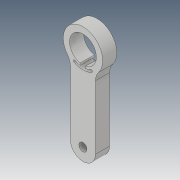
# Autodesk Inventor part: gripperPart4
Saved by Autodesk Inventor 2018 (Build 220112000, 112)
## iProperties
Created: 2020-01-19
Part Number: gripperPart4
Material: Generic
Document SubType Name: Modeling
Designer: anirudh
Density: 1 g/cm^3
Appearance: Default
Author: anirudh
Autodesk Inventor part; units mm, degrees
ref_plane "YZ Plane" through (0, 0, 0) normal (1, 0, 0) x (0, 1, 0)
ref_plane "XZ Plane" through (0, 0, 0) normal (0, 1, 0) x (-1, 0, 0)
ref_plane "XY Plane" through (0, 0, 0) normal (0, 0, 1) x (1, 0, 0)
sketch "Sketch1" plane through (0, 0, 0) normal (0, 0, 1) x (1, 0, 0)
  arc A0 (9.753, 1.6889) -> (9.316, 0.7861) centre (9.5674, 1.2216) ccw
  arc A1 (9.8188, 1.6571) -> (9.316, 0.7861) centre (9.5674, 1.2216) ccw
  arc A2 (17.316, 0.7861) -> (16.816, 1.6522) centre (17.066, 1.2191) ccw
  arc A3 (17.316, 0.7861) -> (16.816, 1.6522) centre (17.066, 1.2191) ccw
  arc A4 (14.5598, 0.8257) -> (16.816, 1.6522) centre (13.316, 7.7143) ccw
  arc A5 (9.316, 0.7861) -> (17.316, 0.7861) centre (13.316, 7.7143) ccw
  arc A6 (9.316, 0.7861) -> (17.316, 0.7861) centre (13.316, 7.7143) ccw
  arc A7 (9.8188, 1.6571) -> (12.0792, 0.8302) centre (13.316, 7.7143) ccw
  arc A8 (14.5598, 0.8257) -> (16.816, 1.6522) centre (13.316, 7.7143) ccw
  line L0 (7.6645, -17.6857) -> (7.6645, 0.8519)
  line L1 (18.9675, -17.6857) -> (18.9675, 0.8519)
  arc A9 (9.316, 0.7861) -> (17.316, 0.7861) centre (13.316, 7.7143) ccw
  line L2 (7.6645, -17.6857) -> (7.6645, -30.3857)
  line L3 (18.9675, -17.6857) -> (18.9675, -30.3857)
  arc A10 (7.6645, -30.3857) -> (18.9675, -30.3857) centre (13.316, -30.3857) ccw
  circle A11 centre (13.316, -30.3857) radius 1.8
  arc A12 (14.5512, 1.7918) -> (12.0808, 1.7918) centre (13.316, 7.7143) ccw
  arc A13 (18.9675, 0.8519) -> (7.6645, 0.8519) centre (13.316, 7.7143) ccw
  arc A14 (12.0792, 0.8302) -> (12.0808, 1.7918) centre (11.769, 1.3115) ccw
  arc A15 (15.3544, 1.0177) -> (15.3587, 1.025) centre (14.863, 1.3115) ccw
  arc A16 (14.5512, 1.7918) -> (14.5598, 0.8257) centre (14.863, 1.3115) ccw
  point P0 (18.0441, 0.8122)
  point P1 (12.5672, 1.7612)
  point P2 (14.0648, 1.7612)
  point P3 (12.5672, 1.7612)
  point P4 (14.0648, 1.7612)
  dimension "d10" = 3.6
  constraints: 36 point on circle, 17 centre point, 8 coincident, 8 end point, 3 vertical, 1 parallel
  measures "d10" diameter of A11
extrude "Extrusion2" add sketch "Sketch1" along normal blind 6.35
fillet "Fillet2" radius 6.35 2 edges at (7.6645, 0.8519, 3.175) (18.9675, 0.8519, 3.175)
body "Solid2"
